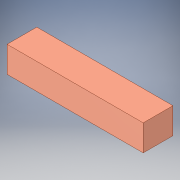
# Autodesk Inventor part: 0207_10
Saved by Autodesk Inventor 2017.3 (Build 213256000, 256)
## iProperties
Part Number: 0207_10
Material: Generisch
Document SubType Name: Modeling
Designer: Nils
Density: 1 g/cm^3
Appearance: 0207_10, 0207_10
Author: Nils
Autodesk Inventor part; units mm, degrees
ref_plane "YZ Plane" through (0, 0, 0) normal (1, 0, 0) x (0, 1, 0)
ref_plane "XZ Plane" through (0, 0, 0) normal (0, 1, 0) x (-1, 0, 0)
ref_plane "XY Plane" through (0, 0, 0) normal (0, 0, 1) x (1, 0, 0)
sketch "0207_10, 0207_10_37" plane through (0, 0, 0) normal (0, 0, 1) x (1, 0, 0)
  line L0 (-5.08, 1.143) -> (5.3848, 1.143)
  line L1 (5.3848, 1.143) -> (5.3848, -1.143)
  line L2 (5.3848, -1.143) -> (-5.08, -1.143)
  line L3 (-5.08, -1.143) -> (-5.08, 1.143)
  constraints: 8 end point
extrude "Extrusion1" add sketch "0207_10, 0207_10_37" along normal blind 2
